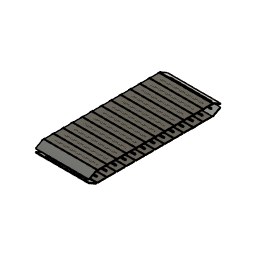
Belt v1 (Autodesk Fusion 360 design; units mm, degrees)
Autodesk Fusion 360 part; units mm, degrees
sketch "Sketch1" plane through (0, 0, 0) normal (0, 0, 1) x (1, 0, 0)
  line L0 (0, 25.032) -> (180, 25.032)
  line L1 (180, 25.032) -> (180, -4.968)
  line L2 (180, -4.968) -> (0, -4.968)
  line L3 (0, -4.968) -> (0, 25.032)
  dimension "d1" = 180
  dimension "d2" = 30
  constraint horizontal L0
  constraint vertical L1
  constraint horizontal L2
  constraint vertical L3
  measures "d1" distance of L0.start L0.end
  measures "d2" distance of L0.start L2.end
extrude "Extrude1" add sketch "Sketch1" along normal blind 2.77 makes body 1
sketch "Sketch2" plane through (0, 0, 0) normal (0, 0, 1) x (1, 0, 0)
  line L0 (21.9257, 8.3236) -> (164.0367, 8.3236)
  line L1 (164.0367, 8.3236) -> (164.0367, 11.9236)
  line L2 (164.0367, 11.9236) -> (21.9257, 11.9236)
  line L3 (21.9257, 11.9236) -> (21.9257, 8.3236)
  dimension "d5" = 3.6
  constraint horizontal L0
  constraint vertical L1
  constraint horizontal L2
  constraint vertical L3
  measures "d5" distance of L0.start L2.end
extrude "Extrude2" add sketch "Sketch2" against normal blind 4.21 bodies 1
chamfer "Chamfer1" distance 1.55 angle 45 2 edges at (92.9812, 11.9236, -4.21) (92.9812, 8.3236, -4.21) on bodies 1
hole "Hole1" at (180, 23.8269, 1.3648) direction (-1, 0, 0) diameter 2 depth 196.9371 tip angle 180 bodies 1
move_face "MoveFace1" to x (1, 0, 0) y (0, 1, 0) z (0, 0, 1) at (1.18, -1.46, 0) 1 faces at (60, 24.6291, 0.7677) on bodies 1
sketch "Sketch3" plane through (0, 0, 0) normal (1, 0, 0) x (0, 1, 0)
  line L0 (-2.6413, 2.7223) -> (-14.8039, 2.7223)
  line L1 (-14.8039, 2.7223) -> (-14.8039, 0.1017)
  line L2 (-14.8039, 0.1017) -> (-2.6413, 0.1017)
  line L3 (-2.6413, 0.1017) -> (-2.6413, 2.7223)
  circle A0 centre (-12.7976, 1.412) radius 1
  circle A1 centre (-5.6973, 1.412) radius 1
  line L4 (-2.6413, 1.412) -> (-14.8039, 1.412)
  dimension "d18" = 2
  dimension "d22" = 2
  constraint horizontal L0
  constraint vertical L1
  constraint horizontal L2
  constraint vertical L3
  constraint midpoint L1 L4.end
  constraint midpoint L3 L4.start
  constraint coincident A1.centre L4
  constraint coincident A0.centre L4
  measures "d18" diameter of A0
  measures "d22" diameter of A1
hole "Hole2" at (0, -3.002, 1.4236) direction (1, 0, 0) diameter 2 depth 199.1 tip angle 180 bodies 1
extrude "Extrude3" add sketch "Sketch3" along normal blind 0.58 separate body contours L0 L1 L3 A0 A1 L4 | L1 L2 L3 A0 A1 L4 makes body 2
move_body "Move2" bodies 2 to x (1, 0, 0) y (0, 1, 0) z (0, 0, 1) at (-1.25, 0, 0)
move_body "Move3" bodies 2 to x (1, 0, 0) y (0, 0.999084, -0.042795) z (0, 0.042795, 0.999084) at (0, -0.0132, -0.5453)
move_body "Move4" bodies 2 to x (1, 0, 0) y (0, 1, 0) z (0, 0, 1) at (0, 3.37, 0.35)
extrude "Extrude4" add 1 faces at (-1.25, 0.0559, 0.8238) along direction (-1, 0, 0) blind 0.1 on bodies 2 bodies 2
extrude "Extrude5" cut 1 faces at (-1.1233, 0.7596, 0.892) along direction (0, -0.999084, 0.042795) blind 0.41 on bodies 2 bodies 2
copy_body "CopyPasteBodies1" bodies 2 makes body 3
move_body "Move5" bodies 3 to x (1, 0, 0) y (0, 1, 0) z (0, 0, 1) at (181.75, 0, 0)
copy_body "Body->Comp1" bodies 2 removing the originals makes body 4 in component "Component"
copy_body "Body->Comp2" bodies 3 removing the originals makes body 5 in component "Component'"
pattern_path "PathPattern1" count 14 spacing 32.4298 from (180, 25.032, 0) along 1 edges at (180, 10.032, 0) of bodies 1 on bodies 1 makes body 6 at (60, -17.3978, 2.77) makes body 7 at (60, -49.8275, 2.77) makes body 8 at (60, -82.2573, 2.77) makes body 9 at (60, -114.6871, 2.77) makes body 10 at (60, -147.1169, 2.77) makes body 11 at (60, -179.5466, 2.77) makes body 12 at (60, -211.9764, 2.77) makes body 13 at (60, -244.4062, 2.77) makes body 14 at (60, -276.8359, 2.77) makes body 15 at (60, -309.2657, 2.77) makes body 16 at (60, -341.6955, 2.77) makes body 17 at (60, -374.1253, 2.77) makes body 18 at (60, -406.555, 2.77)
copy_body "Body->Comp3" bodies 1 removing the originals makes body 19 in component "Component''"
copy_body "CutPasteBodies1" bodies 6 removing the originals makes body 20 in component "Component''"
copy_body "CutPasteBodies2" bodies 7 removing the originals makes body 21 in component "Component''"
move_body "Move1" bodies 4 to x (1, 0, 0) y (0, -1, 0) z (0, 0, -1) at (0, -11.504, 3.2163) in component "Component"
component_pattern "component pattern"
move_body "Move6" bodies 18 to x (1, 0, 0) y (0, 0.891007, 0.45399) z (0, -0.45399, 0.891007) at (0, -42.8928, 181.3909)
move_body "Move2'" bodies 19 to x (1, 0, 0) y (0, 0.866025, -0.5) z (0, 0.5, 0.866025) at (0, -1.114, -1.3103) in component "Component''"
copy_body "CopyPasteBodies2" bodies 13 4 15 5 21 9 18 14 20 16 10 11 17 8 12 19 body 4 seen with x (1, 0, 0) y (0, -0.99912, -0.041931) z (0, 0.041931, -0.99912) at (0, -337.5269, 2.7764) body 5 seen with x (1, 0, 0) y (0, -0.99912, -0.041931) z (0, 0.041931, -0.99912) at (0, -337.5269, 2.7764) makes body 22 makes body 23 makes body 24 makes body 25 makes body 26 makes body 27 makes body 28 makes body 29 makes body 30 makes body 31 makes body 32 makes body 33 makes body 34 makes body 35 makes body 36 makes body 37
move_body "Move7" bodies 22 23 24 25 26 27 28 29 30 31 32 33 34 35 36 37 to x (1, 0, 0) y (0, -1, 0) z (0, 0, -1) at (0.4982, -403.1498, -33.1374)
component "Component'" placed x (1, 0, 0) y (0, -0.99912, -0.041931) z (0, 0.041931, -0.99912) at (0, -12.3269, 2.7764)
component "Component''" placed x (1, 0, 0) y (0, 1, 0) z (0, 0, 1) at (0, 0, 0)
component "Component'" placed x (1, 0, 0) y (0, -0.99912, -0.041931) z (0, 0.041931, -0.99912) at (0, -44.8469, 2.7764)
component "Component'" placed x (1, 0, 0) y (0, -0.99912, -0.041931) z (0, 0.041931, -0.99912) at (0, -77.3669, 2.7764)
component "Component'" placed x (1, 0, 0) y (0, -0.99912, -0.041931) z (0, 0.041931, -0.99912) at (0, -109.8869, 2.7764)
component "Component'" placed x (1, 0, 0) y (0, -0.99912, -0.041931) z (0, 0.041931, -0.99912) at (0, -142.4069, 2.7764)
component "Component'" placed x (1, 0, 0) y (0, -0.99912, -0.041931) z (0, 0.041931, -0.99912) at (0, -174.9269, 2.7764)
component "Component'" placed x (1, 0, 0) y (0, -0.99912, -0.041931) z (0, 0.041931, -0.99912) at (0, -207.4469, 2.7764)
component "Component'" placed x (1, 0, 0) y (0, -0.99912, -0.041931) z (0, 0.041931, -0.99912) at (0, -239.9669, 2.7764)
component "Component'" placed x (1, 0, 0) y (0, -0.99912, -0.041931) z (0, 0.041931, -0.99912) at (0, -272.4869, 2.7764)
component "Component'" placed x (1, 0, 0) y (0, -0.99912, -0.041931) z (0, 0.041931, -0.99912) at (0, -305.0069, 2.7764)
component "Component'" placed x (1, 0, 0) y (0, -0.99912, -0.041931) z (0, 0.041931, -0.99912) at (0, -337.5269, 2.7764)
component "Component'" placed x (1, 0, 0) y (0, -0.99912, -0.041931) z (0, 0.041931, -0.99912) at (0, -370.0469, 2.7764)
component "Component'" placed x (1, 0, 0) y (0, -0.99912, -0.041931) z (0, 0.041931, -0.99912) at (0, -402.5669, 2.7764)
component "Component" placed x (1, 0, 0) y (0, 1, 0) z (0, 0, 1) at (0, 0, 0) in component "Component'"
